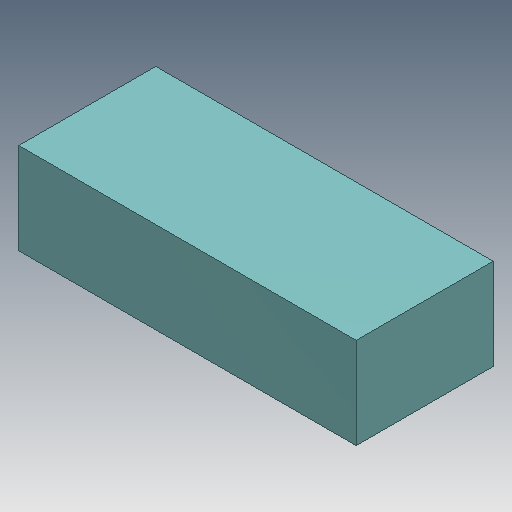
# Autodesk Inventor part: RESONATORSMD
Saved by Autodesk Inventor 2017 (Build 210142000, 142)
## iProperties
Part Number: RESONATORSMD
Material: Generisch
Document SubType Name: Modeling
Designer: Werkstatt
Density: 1 g/cm^3
Appearance: RESONATOR-SMD, RESONATORSMD
Author: Werkstatt
Autodesk Inventor part; units mm, degrees
ref_plane "YZ Plane" through (0, 0, 0) normal (1, 0, 0) x (0, 1, 0)
ref_plane "XZ Plane" through (0, 0, 0) normal (0, 1, 0) x (-1, 0, 0)
ref_plane "XY Plane" through (0, 0, 0) normal (0, 0, 1) x (1, 0, 0)
sketch "RESONATOR-SMD, RESONATORSMD_39" plane through (0, 0, 0) normal (0, 0, 1) x (1, 0, 0)
  line L0 (-1.8, 0.7516) -> (1.9016, 0.7516)
  line L1 (1.9016, 0.7516) -> (1.9016, -0.7516)
  line L2 (1.9016, -0.7516) -> (-1.8, -0.7516)
  line L3 (-1.8, -0.7516) -> (-1.8, 0.7516)
  constraints: 8 end point
extrude "Extrusion1" add sketch "RESONATOR-SMD, RESONATORSMD_39" along normal blind 1
